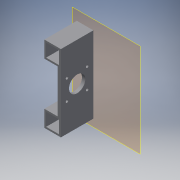
# Autodesk Inventor part: ExtruderMount
Saved by Autodesk Inventor 2016 (Build 200138000, 138)
## iProperties
Created: 2016-05-27
Part Number: ExtruderMount
Material: Generic
Document SubType Name: Modeling
Designer: Scott
Density: 1 g/cm^3
Appearance: Default
Author: Scott
Autodesk Inventor part; units mm, degrees
ref_plane "YZ Plane" through (0, 0, 0) normal (1, 0, 0) x (0, 1, 0)
ref_plane "XZ Plane" through (0, 0, 0) normal (0, 1, 0) x (-1, 0, 0)
ref_plane "XY Plane" through (0, 0, 0) normal (0, 0, 1) x (1, 0, 0)
ref_plane "Work Plane1" through (0, 0, 0) normal (0, 0, 1) x (1, 0, 0)
sketch "Sketch1" plane through (0, 0, 0) normal (0, 0, 1) x (1, 0, 0)
  line L0 (5.0907, -20) -> (5.0907, 0) projected
  line L1 (25.0907, -20) -> (5.0907, -20) projected
  line L2 (25.0907, 0) -> (25.0907, -20) projected
  line L3 (5.0907, 0) -> (25.0907, 0) projected
  line L4 (5.0907, 71.5801) -> (25.0907, 71.5801) projected
  line L5 (5.0907, 91.5801) -> (25.0907, 91.5801) projected
  line L6 (5.0907, 91.5801) -> (5.0907, 71.5801) projected
  line L7 (24.826, 92.0223) -> (24.826, 72.0223) projected
  line L8 (2.3907, 2.7) -> (27.7907, 2.7)
  line L9 (27.7907, 2.7) -> (27.7907, -22.7)
  line L10 (27.7907, -22.7) -> (2.3907, -22.7)
  line L11 (2.3907, -22.7) -> (2.3907, 2.7)
  line L12 (2.3907, 2.7) -> (27.7907, -22.7) construction
  line L13 (27.7907, 2.7) -> (2.3907, -22.7) construction
  line L14 (2.3907, 94.7223) -> (27.7907, 94.7223)
  line L15 (27.7907, 94.7223) -> (27.7907, 69.3223)
  line L16 (27.7907, 69.3223) -> (2.3907, 69.3223)
  line L17 (2.3907, 69.3223) -> (2.3907, 94.7223)
  line L18 (2.3907, 94.7223) -> (27.7907, 69.3223) construction
  line L19 (27.7907, 94.7223) -> (2.3907, 69.3223) construction
  line L20 (25.0907, 72.0223) -> (5.0907, 72.0223)
  line L21 (5.0907, 72.0223) -> (5.0907, 92.0223)
  line L22 (5.0907, 92.0223) -> (25.0907, 92.0223)
  line L23 (25.0907, 92.0223) -> (25.0907, 72.0223)
  line L24 (25.0907, 72.0223) -> (5.0907, 92.0223) construction
  line L25 (5.0907, 72.0223) -> (25.0907, 92.0223) construction
  point P0 (0, 0)
  point P1 (15.0907, -10)
  point P2 (15.0907, 82.0223)
  dimension "d0" = 25.4
  dimension "d1" = 25.4
  dimension "d2" = 25.4
  dimension "d3" = 25.4
  dimension "d4" = 20
  dimension "d5" = 20
  constraints: 36 end point, 6 midpoint, 6 parallel, 3 horizontal, 3 perpendicular
  measures "d0" distance of L9.end L10.end
  measures "d1" distance of L8.end L9.end
  measures "d2" distance of L15.end L16.end
  measures "d3" distance of L14.end L15.end
  measures "d4" distance of L21.end L22.end
  measures "d5" distance of L20.end L21.end
extrude "Extrusion1" add sketch "Sketch1" along normal blind 50
sketch "Sketch2" plane through (27.7907, 69.3223, 0) normal (1, 0, 0) x (0, 0, -1)
  line L0 (0, 25.4) -> (0, 0) projected
  line L1 (0, 25.4) -> (-50, 25.4) projected
  line L2 (-50, 0) -> (-50, 25.4) projected
  line L3 (0, 0) -> (-50, 0) projected
  line L4 (0, -66.6223) -> (0, -92.0223) projected
  line L5 (0, -66.6223) -> (-50, -66.6223) projected
  line L6 (-50, -92.0223) -> (-50, -66.6223) projected
  line L7 (0, -92.0223) -> (-50, -92.0223) projected
  line L8 (0, 25.4) -> (-50, 25.4) projected
  line L9 (0, 25.4) -> (-50, 25.4)
  line L10 (-50, 25.4) -> (-50, -92.0223)
  line L11 (-50, -92.0223) -> (0, -92.0223)
  line L12 (0, -92.0223) -> (0, 25.4)
  point P0 (0, -69.3223)
  constraints: 8 end point, 2 parallel, 1 horizontal, 1 perpendicular
extrude "Extrusion2" add sketch "Sketch2" against normal blind 5.08 contours L12 L5 L10 L3
sketch "Sketch3" plane through (22.7107, 69.3223, 0) normal (-1, 0, 0) x (0, 0, 1)
  line L0 (0, 25.4) -> (0, -92.0223) projected
  line L1 (0, 25.4) -> (50, 25.4) projected
  line L2 (50, -92.0223) -> (50, 25.4) projected
  line L3 (0, -92.0223) -> (50, -92.0223) projected
  circle A0 centre (25, -33.3111) radius 12.5
  line L4 (25, -33.3111) -> (9.5, -33.3111)
  line L5 (9.5, -33.3111) -> (9.5, -48.8111)
  circle A1 centre (9.5, -48.8111) radius 2
  circle A2 centre (9.5, -17.8111) radius 2
  circle A3 centre (40.5, -48.8111) radius 2
  circle A4 centre (40.5, -17.8111) radius 2
  point P0 (0, -69.3223)
  dimension "d10" = 25
  dimension "d11" = 15.5
  dimension "d12" = 15.5
  dimension "d13" = 4
  dimension "d16" = 31
  dimension "d19" = 31
  constraints: 5 centre point, 4 end point, 2 horizontal, 1 coincident, 1 perpendicular, 1 vertical, 6 other
  measures "d10" diameter of A0
  measures "d11" distance of L4.start L4.end
  measures "d12" distance of L4.end L5.end
  measures "d13" diameter of A1
  measures "d16" distance of A1.centre A2.centre
  measures "d19" distance of A1.centre A3.centre
extrude "Extrusion3" cut sketch "Sketch3" against normal blind 5.08 contours A0 | A1 | A2 | A3 | A4
body "Solid1"
